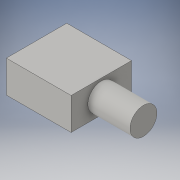
# Autodesk Inventor part: SWITCH
Saved by Autodesk Inventor 2016 (Build 200138000, 138)
## iProperties
Created: 2016-10-04
Part Number: SWITCH
Material: Generic
Document SubType Name: Modeling
Designer: brandn
Density: 1 g/cm^3
Appearance: Default
Author: brandn
Autodesk Inventor part; units mm, degrees
ref_plane "YZ Plane" through (0, 0, 0) normal (1, 0, 0) x (0, 1, 0)
ref_plane "XZ Plane" through (0, 0, 0) normal (0, 1, 0) x (-1, 0, 0)
ref_plane "XY Plane" through (0, 0, 0) normal (0, 0, 1) x (1, 0, 0)
sketch "Sketch1" plane through (0, 0, 0) normal (1, 0, 0) x (0, 1, 0)
  line L0 (1.4781, 6.9278) -> (-5.2783, 6.9278)
  line L1 (-5.2783, 6.9278) -> (-5.2783, -5.823)
  line L2 (-5.2783, -5.823) -> (1.4781, -5.823)
  line L3 (1.4781, -5.823) -> (1.4781, 6.9278)
  point P0 (0, 0)
  dimension "d0" = 12.7508
  dimension "d1" = 6.7564
  constraints: 8 end point, 2 parallel, 1 horizontal, 1 perpendicular
  measures "d0" distance of L2.end L0.start
  measures "d1" distance of L0.start L0.end
extrude "Extrusion1" add sketch "Sketch1" along normal blind 13.6652
sketch "Sketch2" plane through (13.6652, 0, 0) normal (1, 0, 0) x (0, 0, -1)
  point P0 (0, 0)
sketch "Sketch3" plane through (13.6652, 0, 0) normal (1, 0, 0) x (0, 0, -1)
  circle A0 centre (-0.5524, -1.9001) radius 2.8448
  line L0 (-6.9278, 1.4781) -> (-6.9278, -5.2783) projected
  line L1 (-6.9278, -5.2783) -> (5.823, -5.2783) projected
  point P0 (0, 0)
  dimension "d7" = 6.3754
  dimension "d8" = 3.3782
  dimension "d9" = 5.6896
  constraints: 1 centre point
  measures "d7" distance from line of L0 A0.centre
  measures "d8" distance from line of L1 A0.centre
  measures "d9" diameter of A0
extrude "Extrusion2" add sketch "Sketch3" along normal blind 8.89
body "Solid1"
